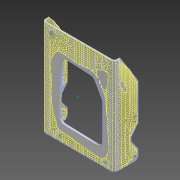
# Autodesk Inventor part: palmrest
Saved by Autodesk Inventor 2018 (Build 220112000, 112)
## iProperties
Created: 2018-07-06
Part Number: palmrest
Material: アルミニウム 6061
Document SubType Name: Sheet Metal
Designer: NaMACHAN
Mass: 46.2587 g
Surface Area: 185.481 cm^2
Volume: 17.1329 cm^3
Density: 2.7 g/cm^3
Sheet Metal Rule: Default
Appearance: アルミニウム - フラット
Flat Pattern Width: 10 cm
Flat Pattern Length: 11.9048 cm
Flat Pattern Area: 119.048 cm^2
Sheet Metal Width: 100.000 mm
Sheet Metal Length: 119.048 mm
Sheet Metal Area: 11904.779 mm^2
Author: NaMACHAN
Autodesk Inventor part; units mm, degrees
ref_plane "YZ Plane" through (0, 0, 0) normal (1, 0, 0) x (0, 1, 0)
ref_plane "XZ Plane" through (0, 0, 0) normal (0, 1, 0) x (-1, 0, 0)
ref_plane "XY Plane" through (0, 0, 0) normal (0, 0, 1) x (1, 0, 0)
sketch "スケッチ1" plane through (0, 0, 0) normal (0, 1, 0) x (-1, 0, 0)
  line L0 (-38, -50) -> (38, -50)
  line L1 (38, -50) -> (38, 50)
  line L2 (38, 50) -> (-38, 50)
  line L3 (-38, 50) -> (-38, -50)
  line L4 (-38, -50) -> (38, 50) construction
  line L5 (38, -50) -> (-38, 50) construction
  point P0 (0, 0)
  dimension "d0" = 76
  dimension "d1" = 100
  measures "d0" distance of L2.end L1.end
  measures "d1" distance of L0.end L1.end
extrude "プレート1" add sketch "スケッチ1" along normal blind 2
sketch "スケッチ2" plane through (36, 0, -50) normal (1, 0, 0) x (0, 1, 0)
  line L0 (0, 100) -> (0, 0)
  line L1 (0, 0) -> (25, 0)
  line L2 (25, 0) -> (25, 100)
  line L3 (25, 100) -> (0, 100)
  constraints: 6 end point, 1 horizontal, 1 perpendicular, 1 vertical
edge flange "フランジ1" height 25 angle 90 thickness 2 bend radius 2 thickness toward (1, 0, 0) relief tear relief width 2 relief depth 1 corner gap 2 corner form 0 edges at (38, 2, 0) (-38, 2, 0) wall of the first edge with corners at (36, 0, 50) (36, 0, -50) (36, 25, -50) (36, 25, 50)
bend "曲げ1"
corner "コーナー1"
sketch "スケッチ3" plane through (38, 25, 50) normal (1, 0, 0) x (0, 0, -1)
  line L0 (0, -21) -> (0, 0) projected
  line L1 (100, 0) -> (100, -21) projected
  line L2 (0, 0) -> (100, 0) projected
  point P0 (50, -25)
  point P1 (60, -4)
  point P2 (96, -4)
  dimension "d14" = 4
  dimension "d15" = 36
  dimension "d16" = 4
  constraints: 1 horizontal alignment
  measures "d14" distance from line of L1 point (96, -4)
  measures "d15" distance of point (60, -4) point (96, -4)
  measures "d16" distance from line of L2 point (96, -4)
hole "穴1" at (38, 21, -10) at (38, 21, -46) direction (-1, 0, 0) diameter 3 end through all
sketch "スケッチ6" plane through (0, 0, 0) normal (0, -1, 0) x (1, 0, 0)
  line L0 (-34, 50) -> (-34, -50) projected
  line L1 (-34, 50) -> (34, 50) projected
  point P0 (0, 0)
  point P1 (-27, 43)
  dimension "d30" = 7
  dimension "d31" = 7
  measures "d30" distance from line of L0 point (-27, 43)
  measures "d31" distance from line of L1 point (-27, 43)
hole "穴2" at (-27, 0, 43) direction (0, 1, 0) diameter 6 end through all
sketch "スケッチ7" plane through (0, 2, 0) normal (0, 1, 0) x (1, 0, 0)
  line L0 (34, -50) -> (-34, -50) projected
  line L1 (-34, 50) -> (-34, -50) projected
  line L2 (34, -50) -> (34, 50) projected
  line L3 (-34, 50) -> (34, 50) projected
  point P0 (0, 0)
  point P1 (29, -45)
  point P2 (-19, -45)
  point P3 (-19, 45)
  point P4 (29, 45)
  dimension "d46" = 5
  dimension "d47" = 15
  dimension "d48" = 5
  dimension "d49" = 5
  constraints: 2 horizontal alignment, 2 vertical alignment
  measures "d46" distance from line of L0 point (29, -45)
  measures "d47" distance from line of L1 point (-19, -45)
  measures "d48" distance from line of L2 point (29, -45)
  measures "d49" distance from line of L3 point (-19, 45)
hole "穴3" at (29, 2, 45) at (-19, 2, 45) at (-19, 2, -45) at (29, 2, -45) direction (0, -1, 0) diameter 3 end through all
sketch "スケッチ8" plane through (0, 0, 0) normal (0, -1, 0) x (1, 0, 0)
  point P0 (0, 0)
sketch "スケッチ9" plane through (38, 25, 50) normal (1, 0, 0) x (0, 0, -1)
  line L0 (90.3208, 0) -> (80.3701, -7.3419)
  line L1 (80.3701, -7.3419) -> (76.2406, -7.3419)
  line L2 (76.2406, -7.3419) -> (66.8372, 0)
  line L3 (0, 0) -> (100, 0) projected
  line L4 (90.3208, 0) -> (66.8372, 0)
  line L5 (28.7234, 0) -> (0, -18.0779)
  line L6 (0, -21) -> (0, 0) projected
  line L7 (0, -18.0779) -> (0, 0)
  line L8 (0, 0) -> (28.7234, 0)
  point P0 (50, -25)
  constraints: 14 end point, 3 point on line, 2 collinear, 1 horizontal, 1 perpendicular
extrude "押し出し3" cut sketch "スケッチ9" against normal blind 100
sketch "スケッチ10" plane through (0, 0, 0) normal (0, -1, 0) x (1, 0, 0)
  line L0 (16.2167, 26.1367) -> (25.582, 9.0798)
  line L1 (25.582, 9.0798) -> (25.582, -34.0132)
  line L2 (25.582, -34.0132) -> (-20.3935, -32.572)
  line L3 (-20.3935, -32.572) -> (-17.0787, 27.96)
  line L4 (-17.0787, 27.96) -> (16.2167, 26.1367)
  point P0 (0, 0)
  constraints: 10 end point, 1 perpendicular, 1 point on line, 1 vertical
extrude "押し出し4" cut sketch "スケッチ10" against normal blind 100
fillet "コーナーR3" radius 6 5 edges at (25.582, 1, -34.0132) (25.582, 1, 9.0798) (16.2167, 1, 26.1367) (-17.0787, 1, 27.96) (-20.3935, 1, -32.572)
fillet "コーナーR4" radius 4 1 edges at (37, 25, -50)
fillet "コーナーR5" radius 4 1 edges at (-37, 25, -50)
equation "\"d22\" = Thickness"
equation "\"d37\" = Thickness"
equation "\"d44\" = Thickness"
equation "\"d2\" = Thickness"
equation "\"d3\" = BendReliefWidth"
equation "\"d4\" = BendReliefDepth"
equation "\"d5\" = MinimumRemnant"
equation "\"d6\" = TransitionRadius"
equation "\"d9\" = BendRadius"
equation "\"d10\" = CornerReliefSize"
equation "\"d11\" = GapSize"
equation "\"d12\" = JacobiRadiusSize"
equation "\"BendRadius\" = Thickness"
equation "\"BendReliefWidth\" = Thickness"
equation "\"BendReliefDepth\" = 0.5 * Thickness"
equation "\"CornerReliefSize\" = 4 * Thickness"
equation "\"MinimumRemnant\" = 2 * Thickness"
equation "\"TransitionRadius\" = BendRadius"
equation "\"JacobiRadiusSize\" = Thickness"
equation "\"GapSize\" = Thickness"
equation "\"Thickness\" = 2"
